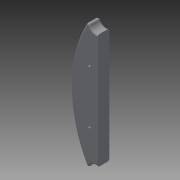
# Autodesk Inventor part: naraznik_kryt
Saved by Autodesk Inventor 2015 (Build 190159000, 159)
## iProperties
Created: 2015-01-01
Part Number: naraznik_kryt
Material: Generic
Document SubType Name: Modeling
Designer: Turboslimak
Density: 1 g/cm^3
Appearance: Default
Author: Turboslimak
Autodesk Inventor part; units mm, degrees
ref_plane "YZ Plane" through (0, 0, 0) normal (1, 0, 0) x (0, 1, 0)
ref_plane "XZ Plane" through (0, 0, 0) normal (0, 1, 0) x (-1, 0, 0)
ref_plane "XY Plane" through (0, 0, 0) normal (0, 0, 1) x (1, 0, 0)
sketch "Sketch1" plane through (0, 0, 0) normal (0, 1, 0) x (-1, 0, 0)
  line L0 (-10.5, 65.5) -> (-10.5, -65.5)
  line L1 (-10.5, 65.5) -> (-10.5, -65.5)
  line L2 (-10.5, -65.5) -> (-10.5, 65.5)
  line L3 (-10.5, -65.5) -> (-10.5, -30.5)
  line L4 (-10.5, 65.5) -> (-10.5, 30.15)
  line L5 (-10.5, 30.5) -> (-10.5, -30.5)
  line L6 (-10.5, 30.5) -> (-10.5, -30.5)
  circle A0 centre (-0.5, -30.5) radius 1.5
  line L7 (-10.5, -30.5) -> (-10.5, 30.15)
  circle A1 centre (-0.5, 30.15) radius 1.5
  line L8 (-10.5, -0.175) -> (20.5, -0.175)
  line L9 (-10.5, -0.175) -> (-10.5, -65.675)
  line L10 (-10.5, -0.175) -> (-10.5, 65.325)
  arc A2 (-10.5, 65.325) -> (-0.2045, 74.8119) centre (-7.9767, 72.9166) ccw
  arc A3 (-0.2045, -75.1619) -> (-10.5, -65.675) centre (-7.9767, -73.2666) ccw
  arc A4 (-0.2045, -75.1619) -> (-0.2045, 74.8119) centre (-125.6452, -0.175) ccw
  line L11 (-10.5, -65.675) -> (-10.5, 65.325)
  point P0 (0, 0)
  dimension "d13" = 35
  dimension "d14" = 35.35
  dimension "d17" = 3
  dimension "d21" = 3
  dimension "d24" = 31
  dimension "d27" = 65.5
  dimension "d28" = 65.5
  dimension "d35" = 14
  dimension "d36" = 8
  dimension "d37" = 14
  dimension "d38" = 8
  constraints: 24 end point, 7 point on circle, 5 centre point, 2 point on line, 1 horizontal, 1 midpoint, 1 vertical
  measures "d13" distance of L2.start L3.end
  measures "d14" distance of L0.start L4.end
  measures "d17" diameter of A0
  measures "d21" diameter of A1
  measures "d24" distance of L8.start L8.end
  measures "d27" distance of L8.start L9.end
  measures "d28" distance of L8.start L10.end
  measures "d35" distance of L11.end A2.end
  measures "d36" radius of A2
  measures "d37" distance of L9.end A3.start
  measures "d38" radius of A3
extrude "Extrusion5" add sketch "Sketch1" along normal blind 13
fillet "Fillet1" radius 2 2 edges at (0.2045, 6.5, 74.8119) (0.2045, 6.5, -75.1619)
fillet "Fillet2" radius 2 12 edges at (-16.0052, 0, -36.1415) (-16.0052, 0, 35.7915) (-0.9895, 0, 70.5908) (4.8517, 0, 65.5522) (-0.9895, 0, -70.9408) (4.8517, 0, -65.9022) (-0.9895, 13, 70.5908) (4.8517, 13, 65.5522) (-0.9895, 13, -70.9408) (4.8517, 13, -65.9022) (-16.0052, 13, -36.1415) (-16.0052, 13, 35.7915)
body "Solid3"
